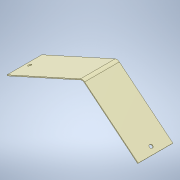
# Autodesk Inventor part: クランクガード
Saved by Autodesk Inventor 2020.2 (Build 242310000, 310)
## iProperties
Created: 2020-03-30
Part Number: クランクガード
Material: ポリプロピレン
Document SubType Name: Modeling
Designer: aoyama
Density: 0.899 g/cm^3
Appearance: 滑らか - 灰色
Author: aoyama
Autodesk Inventor part; units mm, degrees
ref_plane "YZ Plane" through (0, 0, 0) normal (1, 0, 0) x (0, 1, 0)
ref_plane "XZ Plane" through (0, 0, 0) normal (0, 1, 0) x (-1, 0, 0)
ref_plane "XY Plane" through (0, 0, 0) normal (0, 0, 1) x (1, 0, 0)
sketch "スケッチ1" plane through (0, 0, 0) normal (0, 0, 1) x (1, 0, 0)
  circle A0 centre (-56.2051, 45.5451) radius 2.75
  arc A1 (8.9566, 76.3281) -> (6.09, 76.7004) centre (7.222, 74.1942) ccw
  circle A2 centre (57.2805, 33.1812) radius 3
  line L0 (-57.3371, 48.0513) -> (6.09, 76.7004)
  line L1 (8.9566, 76.3281) -> (59.1728, 35.5091)
  line L2 (-57.6459, 48.7348) -> (5.7812, 77.3839)
  arc A3 (6.09, 76.7004) -> (8.9566, 76.3281) centre (7.222, 74.1942) ccw
  arc A4 (9.4296, 76.9101) -> (5.7812, 77.3839) centre (7.222, 74.1942) ccw
  line L3 (9.4296, 76.9101) -> (59.6459, 36.0911)
  line L4 (-57.6459, 48.7348) -> (-56.2051, 45.5451)
  line L5 (57.2805, 33.1812) -> (59.6459, 36.0911)
  line L6 (-53.0891, 50.793) -> (-52.7804, 50.1095)
  line L7 (55.2929, 38.663) -> (55.766, 39.2449)
  point P0 (0, 0)
  point P1 (5.7812, 77.3839)
  dimension "d0" = 0.75
  dimension "d1" = 0.75
  dimension "d2" = 0.75
  dimension "d3" = 5
  dimension "d4" = 5
  constraints: 16 end point, 6 point on circle, 5 point on line, 3 centre point, 3 perpendicular, 2 parallel, 2 tangent, 12 other
  measures "d0" distance between parallel lines of L0 L2
  measures "d1" radial gap between concentric circles of A1 A4
  measures "d2" distance between parallel lines of L1 L3
  measures "d3" distance between parallel lines of L6 L4
  measures "d4" distance between parallel lines of L5 L7
extrude "押し出し1" add sketch "スケッチ1" along normal blind 30 contours L4 L2 L6 L0 | L6 L2 A4 L3 L7 L1 A1 L0
sketch "スケッチ2" plane through (-57.6459, 48.7348, 30) normal (-0.4116, 0.9113, 0) x (0.9113, 0.4116, 0)
  line L0 (69.5972, 30) -> (0, 30) projected
  line L1 (0, 30) -> (0, 0) projected
  line L2 (69.5972, 0) -> (0, 0) projected
  line L3 (69.5972, 30) -> (69.5972, 0) projected
  circle A0 centre (5, 15) radius 1.5
  point P0 (32.474, 30)
  dimension "d7" = 3
  dimension "d8" = 15
  dimension "d9" = 5
  constraints: 1 centre point
  measures "d7" diameter of A0
  measures "d8" distance from line of L0 A0.centre
  measures "d9" distance from line of L1 A0.centre
extrude "押し出し2" cut sketch "スケッチ2" against normal blind 0.75 contours A0
sketch "スケッチ3" plane through (9.4296, 76.9101, 30) normal (0.6308, 0.776, 0) x (0.776, -0.6308, 0)
  line L0 (59.7137, 30) -> (0, 30) projected
  line L1 (0, 30) -> (0, 0) projected
  line L2 (59.7137, 0) -> (0, 0) projected
  line L3 (59.7137, 30) -> (59.7137, 0) projected
  circle A0 centre (54.7137, 15) radius 1.5
  point P0 (41.1949, 30)
  dimension "d12" = 3
  dimension "d13" = 15
  dimension "d14" = 5
  constraints: 1 centre point
  measures "d12" diameter of A0
  measures "d13" distance from line of L0 A0.centre
  measures "d14" distance from line of L3 A0.centre
extrude "押し出し3" cut sketch "スケッチ3" against normal blind 0.75 contours A0
